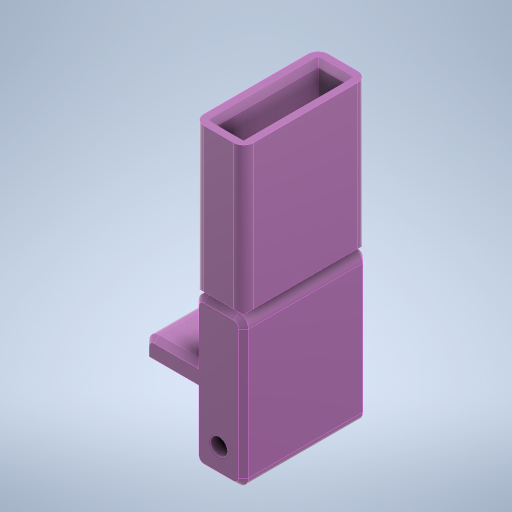
# Autodesk Inventor part: BaseAux_Sensor_V2
Saved by Autodesk Inventor 2024 (Build 280153000, 153)
## iProperties
Created: 2023-11-09
Part Number: BaseAux_Sensor_V2
Material: Generic
Document SubType Name: Modeling
Designer: fredy
Density: 1 g/cm^3
Appearance: Smooth - Purple
Author: fredy
Autodesk Inventor part; units mm, degrees
ref_plane "YZ Plane" through (0, 0, 0) normal (1, 0, 0) x (0, 1, 0)
ref_plane "XZ Plane" through (0, 0, 0) normal (0, 1, 0) x (-1, 0, 0)
ref_plane "XY Plane" through (0, 0, 0) normal (0, 0, 1) x (1, 0, 0)
sketch "Sketch1" plane through (0, 0, 0) normal (0, 0, 1) x (1, 0, 0)
  line L0 (-20, 13.2) -> (-10, 13.2)
  line L1 (-10, 13.2) -> (-10, 0)
  line L2 (-10, 0) -> (0, 0)
  line L3 (0, 0) -> (0, 18)
  line L4 (0, 18) -> (-20, 18)
  line L5 (-20, 18) -> (-20, 13.2)
  point P0 (-10, 6.6)
  dimension "d0" = 18
  dimension "d1" = 20
  dimension "d3" = 10
  dimension "d4" = 4.8
  constraints: 12 end point, 3 horizontal, 2 vertical, 1 coincident, 1 midpoint, 1 perpendicular
  measures "d0" distance of L2.end L3.end
  measures "d1" distance of L3.end L4.end
  measures "d3" distance of L1.end L2.end
  measures "d4" distance of L4.end L0.start
extrude "Extrusion1" add sketch "Sketch1" along normal blind 25
sketch "Sketch4" plane through (-20, 18, 0) normal (0, 1, 0) x (1, 0, 0)
  line L0 (20, 0) -> (10, 0)
  line L1 (10, 0) -> (10, -25)
  line L2 (10, -25) -> (20, -25)
  line L3 (20, -25) -> (20, 0)
  line L4 (0, 0) -> (0, -25) projected
  line L5 (0, -12.5) -> (20, -12.5)
  circle A0 centre (15, -6.5) radius 3.05
  circle A1 centre (15, -18.5) radius 3.05
  dimension "d21" = 10
  dimension "d25" = 12
  dimension "d26" = 6.1
  dimension "d27" = 5
  constraints: 10 end point, 2 centre point, 2 coincident, 2 midpoint, 2 parallel, 1 horizontal, 1 perpendicular, 1 symmetric about line, 1 other
  measures "d21" distance between parallel lines of L3 L1
  measures "d25" diameter of A0.centre L5
  measures "d26" diameter of A1
  measures "d27" distance from line of L3 A0.centre
extrude "Extrusion2" add sketch "Sketch4" along normal blind 12
sketch "Sketch2" plane through (0, 0, 25) normal (0, 0, 1) x (1, 0, 0)
  line L0 (-10, 0) -> (0, 0) construction
  line L1 (-5, 0) -> (-5, 18) construction
  line L2 (0, 18) -> (-20, 18) construction
  line L3 (-10, 13.2) -> (-10, 0) construction
  line L4 (-10, 5.5) -> (0, 5.5) construction
  point P0 (-5, 5.5)
  dimension "d15" = 12.5
  constraints: 4 end point, 3 point on line, 2 midpoint, 1 perpendicular, 1 vertical
  measures "d15" distance between parallel lines of L2 L4
hole "Hole1" at (-5, 5.5, 25) direction (0, 0, -1) diameter 3.475 end through all
fillet "Fillet3" radius 2 5 edges at (-20, 18, 12.5) (-10, 0, 12.5) (0, 0, 12.5) (0, 30, 12.5) (-10, 30, 12.5)
chamfer "Chamfer2" distance 1 angle 45 26 edges at (-14, 18, 25) (-19.4142, 17.4142, 25) (-20, 14.6, 25) (-15, 13.2, 25) (-10, 23, 25) (-9.4142, 29.4142, 25) (-5, 30, 25) (-0.5858, 29.4142, 25) (0, 15, 25) (-0.5858, 0.5858, 25) (-5, 0, 25) (-9.4142, 0.5858, 25) (-10, 7.6, 25) (-0.5858, 0.5858, 0) (0, 15, 0) (-0.5858, 29.4142, 0) (-5, 30, 0) (-9.4142, 29.4142, 0) (-10, 23, 0) (-5, 0, 0) (-9.4142, 0.5858, 0) (-10, 7.6, 0) (-15, 13.2, 0) (-14, 18, 0) (-19.4142, 17.4142, 0) (-20, 14.6, 0)
sketch "Sketch5" plane through (-20, 30, 0) normal (0, 1, 0) x (1, 0, 0)
  line L0 (10, -1) -> (10, -24) projected
  line L1 (20, -24) -> (20, -1) projected
  line L2 (18, 0) -> (12, 0) projected
  line L3 (12, -25) -> (18, -25) projected
  line L4 (10, 0) -> (20, 0)
  line L5 (20, 0) -> (20, -25)
  line L6 (20, -25) -> (10, -25)
  line L7 (10, -25) -> (10, 0)
  point P0 (20, 0)
  point P1 (20, -12.5)
  point P2 (10, -12.5)
  point P3 (15, 0)
  point P4 (15, -25)
  point P5 (20, -1)
  point P6 (18, 0)
  constraints: 8 end point, 4 midpoint, 2 horizontal alignment, 2 parallel, 2 vertical alignment, 1 horizontal, 1 perpendicular
extrude "Extrusion3" add sketch "Sketch5" along normal blind 30 separate body
extrude "Extrusion4" cut sketch "Sketch4" along normal blind 20 contours A0 | A1 bodies 2
sketch "Sketch6" plane through (-20, 60, 0) normal (0, 1, 0) x (1, 0, 0)
  line L0 (12.35, -2.35) -> (17.65, -2.35)
  line L1 (17.65, -2.35) -> (17.65, -22.65)
  line L2 (17.65, -22.65) -> (12.35, -22.65)
  line L3 (12.35, -22.65) -> (12.35, -2.35)
  line L4 (20, -25) -> (20, 0) projected
  line L5 (10, -25) -> (20, -25) projected
  point P0 (17.65, -12.5)
  point P1 (20, -12.5)
  point P2 (15, -22.65)
  point P3 (15, -25)
  dimension "d38" = 20.3
  dimension "d39" = 5.3
  constraints: 8 end point, 4 midpoint, 2 parallel, 1 horizontal, 1 horizontal alignment, 1 perpendicular, 1 vertical alignment
  measures "d38" distance of L0.end L1.end
  measures "d39" distance of L0.start L0.end
extrude "Extrusion5" cut sketch "Sketch6" against normal blind 20 bodies 2
chamfer "Chamfer3" distance 1 angle 45 4 edges at (-10, 30, 12.5) (-5, 30, 0) (0, 30, 12.5) (-5, 30, 25)
chamfer "Chamfer4" distance 1 angle 45 4 edges at (-7.65, 60, 12.5) (-5, 60, 22.65) (-2.35, 60, 12.5) (-5, 60, 2.35)
fillet "Fillet4" radius 2 4 edges at (-10, 45.5, 25) (0, 45.5, 25) (0, 45.5, 0) (-10, 45.5, 0)
